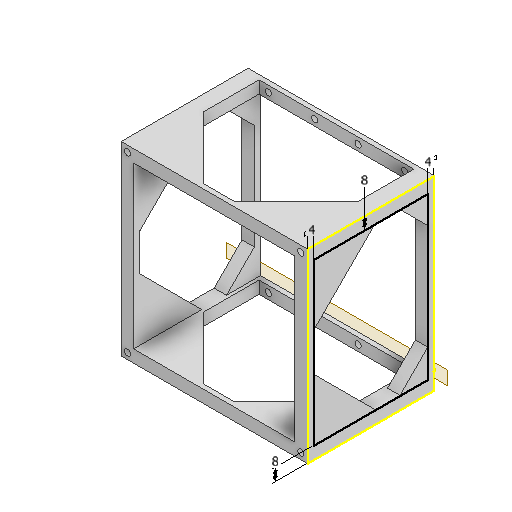
# Autodesk Inventor part: 160mm_shunt_box
Saved by Autodesk Inventor 2023 (Build 270158000, 158)
## iProperties
Created: 2021-07-06
Part Number: 160mm_shunt_box
Material: Generic
Document SubType Name: Modeling
Designer: CDT
Density: 1 g/cm^3
Appearance: Default
Author: CDT
Autodesk Inventor part; units mm, degrees
ref_plane "YZ Plane" through (0, 0, 0) normal (1, 0, 0) x (0, 1, 0)
ref_plane "XZ Plane" through (0, 0, 0) normal (0, 1, 0) x (-1, 0, 0)
ref_plane "XY Plane" through (0, 0, 0) normal (0, 0, 1) x (1, 0, 0)
ref_plane "Work Plane1" through (0, 0, 0) normal (0, 0, 1) x (1, 0, 0)
sketch "Sketch1" plane through (0, 0, 0) normal (0, 0, 1) x (1, 0, 0)
  line L0 (62.5078, -11.1378) -> (-57.4922, -11.1378)
  line L1 (-57.4922, -11.1378) -> (-57.4922, 108.8622)
  line L2 (-57.4922, 108.8622) -> (62.5078, 108.8622)
  line L3 (62.5078, 108.8622) -> (62.5078, -11.1378)
  line L4 (-57.4922, -11.1378) -> (-49.4922, -11.1378)
  line L5 (-49.4922, -11.1378) -> (-49.4922, -3.1378)
  line L6 (-49.4922, -3.1378) -> (-57.4922, -3.1378)
  line L7 (-57.4922, -3.1378) -> (-57.4922, -11.1378)
  line L8 (-57.4922, 108.8622) -> (-49.4922, 108.8622)
  line L9 (-49.4922, 108.8622) -> (-49.4922, 100.8622)
  line L10 (-49.4922, 100.8622) -> (-57.4922, 100.8622)
  line L11 (-57.4922, 100.8622) -> (-57.4922, 108.8622)
  line L12 (62.5078, -11.1378) -> (54.5078, -11.1378)
  line L13 (54.5078, -11.1378) -> (54.5078, -3.1378)
  line L14 (54.5078, -3.1378) -> (62.5078, -3.1378)
  line L15 (62.5078, -3.1378) -> (62.5078, -11.1378)
  line L16 (62.5078, 108.8622) -> (54.5078, 108.8622)
  line L17 (54.5078, 108.8622) -> (54.5078, 100.8622)
  line L18 (54.5078, 100.8622) -> (62.5078, 100.8622)
  line L19 (62.5078, 100.8622) -> (62.5078, 108.8622)
  circle A0 centre (-53.4922, -7.1378) radius 2
  circle A1 centre (-53.4922, 104.8622) radius 2
  circle A2 centre (58.5078, -7.1378) radius 2
  circle A3 centre (58.5078, 104.8622) radius 2
  line L20 (-49.4922, -3.1378) -> (54.5078, -3.1378)
  line L21 (54.5078, -3.1378) -> (54.5078, 100.8622)
  line L22 (54.5078, 100.8622) -> (-49.4922, 100.8622)
  line L23 (-49.4922, 100.8622) -> (-49.4922, -3.1378)
  point P0 (0, 0)
  point P1 (54.5078, -3.1378)
  point P2 (-49.4922, -3.1378)
  point P3 (-49.4922, -3.1378)
  point P4 (54.5078, 100.8622)
  point P5 (54.5078, 100.8622)
  point P6 (54.5078, -3.1378)
  dimension "d0" = 120
  dimension "d1" = 120
  dimension "d2" = 8
  dimension "d3" = 8
  dimension "d4" = 8
  dimension "d5" = 8
  dimension "d6" = 8
  dimension "d7" = 8
  dimension "d8" = 8
  dimension "d9" = 8
  dimension "d10" = 4
  dimension "d11" = 4
  dimension "d12" = 4
  dimension "d13" = 4
  dimension "d14" = 4
  dimension "d15" = 4
  dimension "d16" = 4
  dimension "d17" = 4
  dimension "d18" = 4
  dimension "d19" = 4
  dimension "d20" = 4
  dimension "d21" = 4
  dimension "d22" = 8
  dimension "d23" = 8
  dimension "d24" = 8
  dimension "d25" = 8
  constraints: 48 end point, 12 parallel, 6 horizontal, 6 perpendicular, 4 centre point
  measures "d0" distance of L1.end L2.end
  measures "d1" distance of L0.end L1.end
  measures "d2" distance of L6.end L5.end
  measures "d3" distance of L5.end L4.end
  measures "d4" distance of L9.end L10.end
  measures "d5" distance of L8.end L9.end
  measures "d6" distance of L13.end L14.end
  measures "d7" distance of L12.end L13.end
  measures "d8" distance of L18.end L17.end
  measures "d9" distance of L17.end L16.end
  measures "d10" diameter of A0
  measures "d11" diameter of A1
  measures "d12" diameter of A2
  measures "d13" diameter of A3
  measures "d14" distance from line of L0 A2.centre
  measures "d15" distance from line of L3 A2.centre
  measures "d16" distance from line of L2 A3.centre
  measures "d17" distance from line of L3 A3.centre
  measures "d18" distance from line of L2 A1.centre
  measures "d19" distance from line of L1 A1.centre
  measures "d20" distance from line of L1 A0.centre
  measures "d21" distance from line of L0 A0.centre
  measures "d22" distance between parallel lines of L1 L23
  measures "d23" distance between parallel lines of L2 L22
  measures "d24" distance between parallel lines of L3 L21
  measures "d25" distance between parallel lines of L0 L20
extrude "Extrusion1" add sketch "Sketch1" along normal blind 82 contours L0 L13 L14 L3 | L0 L5 L20 L13 | L14 L21 L18 L3 | L0 L1 L6 L5 | L18 L17 L2 L3 | L6 L1 L10 L23 | L22 L9 L2 L17 | L10 L1 L2 L9
sketch "Sketch2" plane through (62.5078, -11.1378, 0) normal (1, 0, 0) x (0, 0, -1)
  line L0 (-78, 8) -> (-4, 8)
  line L1 (-4, 8) -> (-4, 112)
  line L2 (-4, 112) -> (-78, 112)
  line L3 (-78, 112) -> (-78, 8)
  line L4 (0, 120) -> (-82, 120) projected
  line L5 (-82, 0) -> (-82, 120) projected
  line L6 (0, 0) -> (0, 120) projected
  line L7 (0, 0) -> (-82, 0) projected
  point P0 (0, 11.1378)
  dimension "d30" = 8
  dimension "d31" = 4
  dimension "d67" = 8
  dimension "d68" = 4
  constraints: 8 end point, 2 parallel, 1 horizontal, 1 perpendicular
  measures "d30" distance between parallel lines of L4 L2
  measures "d31" distance between parallel lines of L5 L3
  measures "d67" distance between parallel lines of L7 L0
  measures "d68" distance between parallel lines of L6 L1
extrude "Extrusion2" cut sketch "Sketch2" against normal blind 160 contours L3 L2 L1 L0
sketch "Sketch3" plane through (-57.4922, 108.8622, 0) normal (0, 1, 0) x (1, 0, 0)
  line L0 (110, -79) -> (10, -79)
  line L1 (10, -79) -> (10, -3)
  line L2 (10, -3) -> (110, -3)
  line L3 (110, -3) -> (110, -79)
  line L4 (0, 0) -> (0, -82) projected
  line L5 (120, 0) -> (120, -82) projected
  line L6 (120, -82) -> (0, -82) projected
  line L7 (120, 0) -> (0, 0) projected
  point P0 (57.4922, 0)
  dimension "d38" = 10
  dimension "d39" = 10
  dimension "d40" = 3
  dimension "d41" = 3
  constraints: 8 end point, 2 parallel, 1 horizontal, 1 perpendicular
  measures "d38" distance between parallel lines of L4 L1
  measures "d39" distance between parallel lines of L5 L3
  measures "d40" distance between parallel lines of L6 L0
  measures "d41" distance between parallel lines of L7 L2
extrude "Extrusion3" cut sketch "Sketch3" against normal blind 160 contours L0 L1 L2 L3
sketch "Sketch4" plane through (-47.4922, -3.1378, 3) normal (0, 0, 1) x (1, 0, 0)
  circle A0 centre (94, 108) radius 2
  circle A1 centre (6, 108) radius 2
  circle A2 centre (6, -4) radius 2
  circle A3 centre (94, -4) radius 2
  line L0 (100, -8) -> (0, -8) projected
  line L1 (110, -8) -> (110, 112) projected
  line L2 (-10, 112) -> (-10, -8) projected
  line L3 (110, 112) -> (-10, 112) projected
  circle A4 centre (64, 108) radius 2
  circle A5 centre (64, -4) radius 2
  line L4 (100, 0) -> (100, -8) projected
  circle A6 centre (36, -4) radius 2
  circle A7 centre (36, 108) radius 2
  line L5 (100, 112) -> (100, 104) projected
  line L6 (0, 112) -> (0, 104) projected
  line L7 (0, 0) -> (0, -8) projected
  point P0 (47.4922, 3.1378)
  dimension "d47" = 4
  dimension "d48" = 4
  dimension "d49" = 4
  dimension "d50" = 4
  dimension "d51" = 4
  dimension "d52" = 16
  dimension "d53" = 4
  dimension "d54" = 16
  dimension "d55" = 16
  dimension "d56" = 16
  dimension "d57" = 4
  dimension "d58" = 4
  dimension "d159" = 4
  dimension "d161" = 4
  dimension "d162" = 4
  dimension "d163" = 4
  dimension "d165" = 4
  dimension "d166" = 4
  dimension "d169" = 4
  dimension "d170" = 4
  dimension "d171" = 46
  dimension "d172" = 46
  dimension "d173" = 46
  dimension "d174" = 46
  constraints: 8 centre point
  measures "d47" diameter of A0
  measures "d48" diameter of A1
  measures "d49" diameter of A2
  measures "d50" diameter of A3
  measures "d51" distance from line of L0 A3.centre
  measures "d52" distance from line of L1 A3.centre
  measures "d53" distance from line of L0 A2.centre
  measures "d54" distance from line of L2 A2.centre
  measures "d55" distance from line of L2 A1.centre
  measures "d56" distance from line of L1 A0.centre
  measures "d57" distance from line of L3 A0.centre
  measures "d58" distance from line of L3 A1.centre
  measures "d159" diameter of A5
  measures "d161" distance from line of L0 A5.centre
  measures "d162" diameter of A6
  measures "d163" diameter of A7
  measures "d165" distance from line of L3 A4.centre
  measures "d166" distance from line of L3 A7.centre
  measures "d169" distance from line of L0 A6.centre
  measures "d170" diameter of A4
  measures "d171" distance from line of L1 A5.centre
  measures "d172" distance from line of L2 A6.centre
  measures "d173" distance from line of L1 A4.centre
  measures "d174" distance from line of L2 A7.centre
extrude "Extrusion4" cut sketch "Sketch4" against normal through all
chamfer "Chamfer3" distance 40 angle 45 4 edges at (-47.4922, 104.8622, 79) (-47.4922, -7.1378, 79) (52.5078, 104.8622, 79) (52.5078, -7.1378, 79)
chamfer "Chamfer17" distance 18 angle 45 4 edges at (-53.4922, -3.1378, 4) (58.5078, -3.1378, 4) (-53.4922, 100.8622, 4) (58.5078, 100.8622, 4)
chamfer "Chamfer18" distance 40 angle 45 4 edges at (58.5078, -3.1378, 78) (58.5078, 100.8622, 78) (-53.4922, 100.8622, 78) (-53.4922, -3.1378, 78)
equation "\"d25\" = d9"
equation "\"d54\" = d52"
equation "\"d55\" = d52"
equation "\"d56\" = d52"
body "Solid1"
